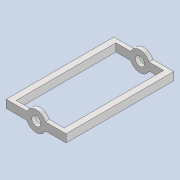
# Autodesk Inventor part: cable_holder_1
Saved by Autodesk Inventor 2020 (Build 240168000, 168)
## iProperties
Created: 2021-07-19
Part Number: cable_holder_1
Material: Generic
Document SubType Name: Modeling
Designer: Shuang Peng
Density: 1 g/cm^3
Appearance: Default
Author: Shuang Peng
Autodesk Inventor part; units mm, degrees
ref_plane "YZ Plane" through (0, 0, 0) normal (1, 0, 0) x (0, 1, 0)
ref_plane "XZ Plane" through (0, 0, 0) normal (0, 1, 0) x (-1, 0, 0)
ref_plane "XY Plane" through (0, 0, 0) normal (0, 0, 1) x (1, 0, 0)
sketch "Sketch1" plane through (0, 0, 0) normal (0, 0, 1) x (1, 0, 0)
  circle A0 centre (0, 0) radius 5
  line L0 (-15, 2) -> (-15, -2)
  line L1 (-15, -2) -> (15, -2)
  line L2 (15, -2) -> (15, 2)
  line L3 (15, 2) -> (-15, 2)
  line L4 (-15, 2) -> (15, -2) construction
  line L5 (-15, -2) -> (15, 2) construction
  point P0 (4.5826, 2)
  point P1 (-4.5826, 2)
  point P2 (-4.5826, -2)
  point P3 (4.5826, -2)
  dimension "d0" = 10
  dimension "d1" = 4
  dimension "d2" = 30
  constraints: 12 end point, 2 midpoint, 2 parallel, 1 centre point, 1 coincident, 1 perpendicular, 1 vertical
  measures "d0" diameter of A0
  measures "d1" distance of L0.start L0.end
  measures "d2" distance of L1.end L0.end
extrude "Extrusion1" add sketch "Sketch1" against normal blind 2
ref_plane "Work Plane1" through (0, 0, -54) normal (0, 0, -1) x (1, 0, 0)
sketch "Sketch2" plane through (0, 0, -54) normal (0, 0, -1) x (1, 0, 0)
  circle A0 centre (0, 0) radius 5
  line L0 (15, 2) -> (15, -2)
  line L1 (15, -2) -> (-15, -2)
  line L2 (-15, -2) -> (-15, 2)
  line L3 (-15, 2) -> (15, 2)
  line L4 (15, 2) -> (-15, -2) construction
  line L5 (15, -2) -> (-15, 2) construction
  point P0 (-4.5826, 2)
  point P1 (-4.5826, -2)
  point P2 (4.5826, -2)
  point P3 (4.5826, 2)
  dimension "d5" = 10
  dimension "d6" = 4
  dimension "d7" = 30
  constraints: 12 end point, 2 midpoint, 2 parallel, 1 centre point, 1 coincident, 1 perpendicular, 1 vertical
  measures "d5" diameter of A0
  measures "d6" distance of L0.start L0.end
  measures "d7" distance of L0.end L1.end
extrude "Extrusion2" add sketch "Sketch2" against normal blind 2
sketch "Sketch3" plane through (4.5826, -2, 0) normal (0, -1, 0) x (1, 0, 0)
  line L0 (0, 0) -> (10.4174, 0) projected
  line L1 (0, 0) -> (0, -2) projected
  line L2 (10.4174, -2) -> (0, -2) projected
  line L3 (10.4174, 0) -> (10.4174, -2) projected
  line L4 (10.4174, -54) -> (0, -54) projected
  line L5 (10.4174, -54) -> (10.4174, -52) projected
  line L6 (0, -52) -> (10.4174, -52) projected
  line L7 (0, -54) -> (0, -52) projected
  line L8 (-9.1652, -54) -> (-19.5826, -54) projected
  line L9 (-9.1652, -54) -> (-9.1652, -52) projected
  line L10 (-19.5826, -52) -> (-9.1652, -52) projected
  line L11 (-19.5826, -54) -> (-19.5826, -52) projected
  line L12 (-19.5826, 0) -> (-9.1652, 0) projected
  line L13 (-19.5826, 0) -> (-19.5826, -2) projected
  line L14 (-9.1652, -2) -> (-19.5826, -2) projected
  line L15 (-9.1652, 0) -> (-9.1652, -2) projected
  line L16 (10.4174, 0) -> (10.4174, -2) projected
  line L17 (10.4174, 0) -> (7.4174, 0)
  line L18 (7.4174, 0) -> (7.4174, -54)
  line L19 (7.4174, -54) -> (10.4174, -54)
  line L20 (10.4174, -54) -> (10.4174, 0)
  line L21 (-19.5826, 0) -> (-19.5826, -2) projected
  line L22 (-19.5826, 0) -> (-16.5826, 0)
  line L23 (-16.5826, 0) -> (-16.5826, -54)
  line L24 (-16.5826, -54) -> (-19.5826, -54)
  line L25 (-19.5826, -54) -> (-19.5826, 0)
  point P0 (-4.5826, 0)
  point P1 (-16.5826, 0)
  point P2 (7.4174, -2)
  point P3 (7.4174, -52)
  dimension "d10" = 3
  dimension "d11" = 54
  dimension "d12" = 3
  dimension "d13" = 54
  constraints: 16 end point, 4 parallel, 2 horizontal, 2 perpendicular
  measures "d10" distance of L19.end L18.end
  measures "d11" distance of L18.end L17.end
  measures "d12" distance of L23.end L24.end
  measures "d13" distance of L22.end L23.end
extrude "Extrusion3" add sketch "Sketch3" against normal up to surface (4 mm away) contours L2 L20 L6 L18 | L8 L11 L10 L23 | L10 L25 L14 L23 | L14 L13 L12 L23
sketch "Sketch4" plane through (0, 0, -54) normal (0, 0, -1) x (-1, 0, 0)
  circle A0 centre (0, 0) radius 2.25
  dimension "d16" = 4.5
  constraints: 1 centre point, 1 coincident
  measures "d16" diameter of A0
extrude "Extrusion4" cut sketch "Sketch4" against normal up to surface (54 mm away)
sketch "Sketch5" plane through (0, 0, 0) normal (0, 0, 1) x (1, 0, 0)
  line L0 (0, 0) -> (-6, 0)
  line L1 (0, 0) -> (6, 0)
  dimension "d19" = 6
  dimension "d20" = 6
  constraints: 4 end point, 2 horizontal
  measures "d19" distance of L0.start L0.end
  measures "d20" distance of L0.start L1.end
hole "Hole1" at (6, 0, 0) at (-6, 0, 0) direction (0, 0, -1) diameter 1.6 depth 100
body "Solid1"
